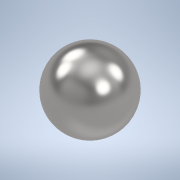
# Autodesk Inventor part: 6138k63_ball
Saved by Autodesk Inventor 2020.1 (Build 241239000, 239)
## iProperties
Created: 2019-10-27
Part Number: 6138k63_ball
Material: Stainless Steel, 440C
Document SubType Name: Modeling
Designer: agmle
Density: 7.75 g/cm^3
Appearance: Semi-Polished
Mass: 0.0248799 g
Surface Area: 0.10524 cm^2
Volume: 0.0032103 cm^3
Author: agmle
Autodesk Inventor part; units mm, degrees
ref_plane "YZ Plane" through (0, 0, 0) normal (1, 0, 0) x (0, 1, 0)
ref_plane "XZ Plane" through (0, 0, 0) normal (0, 1, 0) x (-1, 0, 0)
ref_plane "XY Plane" through (0, 0, 0) normal (0, 0, 1) x (1, 0, 0)
sketch "Sketch1" plane through (0, 0, 0) normal (0, 0, 1) x (1, 0, 0)
  arc A0 (0, -0.9151) -> (0, 0.9151) centre (0, 0) ccw
  line L0 (0, 0.9151) -> (0, -0.9151)
  dimension "d1" = 0.9151
  constraints: 2 coincident, 2 end point, 2 point on circle, 1 centre point, 1 midpoint, 1 vertical
  measures "d1" radius of A0
revolve "Revolution1" add sketch "Sketch1" angle 360 about axis through (0, 0.9151, 0) along (0, -1, 0)
body "Solid1"
